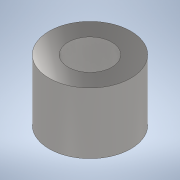
# Autodesk Inventor part: CU-304.5H
Saved by Autodesk Inventor 2020 (Build 240168000, 168)
## iProperties
Created: 2021-09-02
Part Number: CU-304.5H
Material: ステンレス鋼 AISI 304
Document SubType Name: Modeling
Designer: naoki
Density: 8 g/cm^3
Appearance: 半つや出し
Mass: 0.971129 g
Surface Area: 2.1388 cm^2
Volume: 0.121391 cm^3
Author: naoki
Autodesk Inventor part; units mm, degrees
ref_plane "YZ Plane" through (0, 0, 0) normal (1, 0, 0) x (0, 1, 0)
ref_plane "XZ Plane" through (0, 0, 0) normal (0, 1, 0) x (-1, 0, 0)
ref_plane "XY Plane" through (0, 0, 0) normal (0, 0, 1) x (1, 0, 0)
sketch "スケッチ1" plane through (0, 0, 0) normal (0, 0, 1) x (1, 0, 0)
  line L0 (0, 0) -> (3, 0)
  line L1 (3, 0) -> (3, 4.5)
  line L2 (3, 4.5) -> (0, 4.5)
  line L3 (0, 4.5) -> (0, 0)
  line L4 (1.6, 4.5) -> (1.6, 0)
  dimension "d0" = 3
  dimension "d1" = 4.5
  dimension "d2" = 1.6
  constraints: 10 end point, 3 parallel, 2 point on line, 1 horizontal, 1 perpendicular
  measures "d0" distance of L2.end L1.end
  measures "d1" distance of L1.end L0.end
  measures "d2" distance between parallel lines of L3 L4
revolve "回転1" add sketch "スケッチ1" angle 360 about axis through (0, 4.5, 0) along (0, -1, 0) contours L4 L2 L1 L0
